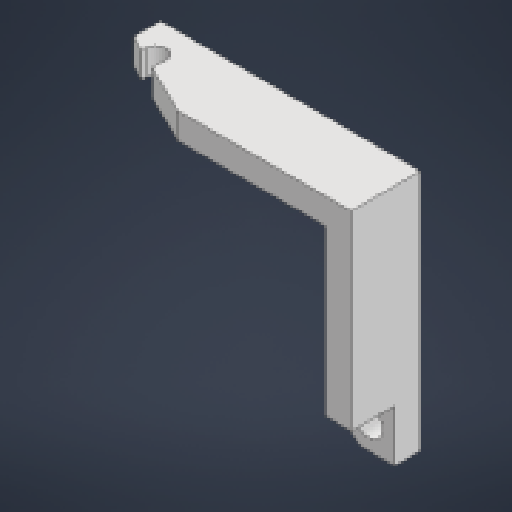
# Autodesk Inventor part: leftfrontwall
Saved by Autodesk Inventor 2026.2 (Build 302298010, 298A)
## iProperties
Created: 2026-09-21
Part Number: leftfrontwall
Material: Generic
Document SubType Name: Modeling
Designer: karol
Density: 1 g/cm^3
Appearance: Default
Author: karol
Autodesk Inventor part; units mm, degrees
ref_plane "YZ Plane" through (0, 0, 0) normal (1, 0, 0) x (0, 1, 0)
ref_plane "XZ Plane" through (0, 0, 0) normal (0, 1, 0) x (-1, 0, 0)
ref_plane "XY Plane" through (0, 0, 0) normal (0, 0, 1) x (1, 0, 0)
sketch "Sketch1" plane through (0, 0, 0) normal (0, 0, 1) x (1, 0, 0)
  line L0 (-58, -60) -> (-60, -60) projected
  line L1 (-60, -60) -> (-60, -39.5) projected
  line L2 (-60, -39.5) -> (-58, -39.5) projected
  line L3 (-58, -39.5) -> (-58, -60) projected
  line L4 (49.6, 30) -> (51.6, 30) projected
  line L5 (51.6, 30) -> (51.6, 9.5) projected
  line L6 (51.6, 9.5) -> (49.6, 9.5) projected
  line L7 (49.6, 9.5) -> (49.6, 30) projected
  line L8 (-58, 39.5) -> (-60, 39.5) projected
  line L9 (-60, 39.5) -> (-60, 60) projected
  line L10 (-60, 60) -> (-58, 60) projected
  line L11 (-58, 60) -> (-58, 39.5) projected
  line L12 (-21.6, -39.5) -> (-19.6, -39.5) projected
  line L13 (-19.6, -39.5) -> (-19.6, -60) projected
  line L14 (-19.6, -60) -> (-21.6, -60) projected
  line L15 (-21.6, -60) -> (-21.6, -39.5) projected
  line L16 (51.6, -30) -> (49.6, -30) projected
  line L17 (49.6, -30) -> (49.6, -9.5) projected
  line L18 (49.6, -9.5) -> (51.6, -9.5) projected
  line L19 (51.6, -9.5) -> (51.6, -30) projected
  line L20 (-21.6, 60) -> (-19.6, 60) projected
  line L21 (-19.6, 60) -> (-19.6, 39.5) projected
  line L22 (-19.6, 39.5) -> (-21.6, 39.5) projected
  line L23 (-21.6, 39.5) -> (-21.6, 60) projected
  line L24 (90, -35) -> (90, 35) projected
  line L25 (90, 35) -> (49.6, 35) projected
  line L26 (49.6, 35) -> (49.6, 60) projected
  line L27 (49.6, 60) -> (90, 60) projected
  line L28 (90, 60) -> (90, 90) projected
  line L29 (90, 90) -> (-19.6, 90) projected
  line L30 (-19.6, 90) -> (-19.6, 65) projected
  line L31 (-19.6, 65) -> (-60, 65) projected
  line L32 (-60, 65) -> (-60, 90) projected
  line L33 (-60, 90) -> (-90, 90) projected
  line L34 (-90, 90) -> (-90, -90) projected
  line L35 (-90, -90) -> (-60, -90) projected
  line L36 (-60, -90) -> (-60, -65) projected
  line L37 (-60, -65) -> (-19.6, -65) projected
  line L38 (-19.6, -65) -> (-19.6, -90) projected
  line L39 (-19.6, -90) -> (90, -90) projected
  line L40 (90, -90) -> (90, -60) projected
  line L41 (90, -60) -> (49.6, -60) projected
  line L42 (49.6, -60) -> (49.6, -35) projected
  line L43 (49.6, -35) -> (90, -35) projected
  line L44 (86, -32) -> (73.8, -32) projected
  line L45 (73.8, -32) -> (73.8, -7.5) projected
  line L46 (73.8, -7.5) -> (86, -7.5) projected
  line L47 (86, -7.5) -> (86, -32) projected
  line L48 (65.8, -32) -> (53.6, -32) projected
  line L49 (53.6, -32) -> (53.6, -7.5) projected
  line L50 (53.6, -7.5) -> (65.8, -7.5) projected
  line L51 (65.8, -7.5) -> (65.8, -32) projected
  line L52 (86, -86) -> (70.6, -86) projected
  line L53 (70.6, -86) -> (70.6, -69.8) projected
  line L54 (70.6, -69.8) -> (86, -69.8) projected
  line L55 (86, -69.8) -> (86, -86) projected
  line L56 (86, 86) -> (86, 69.8) projected
  line L57 (86, 69.8) -> (70.6, 69.8) projected
  line L58 (70.6, 69.8) -> (70.6, 86) projected
  line L59 (70.6, 86) -> (86, 86) projected
  line L60 (73.8, 32) -> (86, 32) projected
  line L61 (86, 32) -> (86, 7.5) projected
  line L62 (86, 7.5) -> (73.8, 7.5) projected
  line L63 (73.8, 7.5) -> (73.8, 32) projected
  line L64 (65.8, 32) -> (65.8, 7.5) projected
  line L65 (65.8, 7.5) -> (53.6, 7.5) projected
  line L66 (53.6, 7.5) -> (53.6, 32) projected
  line L67 (53.6, 32) -> (65.8, 32) projected
  line L68 (-69.6, -87) -> (-85, -87) projected
  line L69 (-85, -87) -> (-85, -70.8) projected
  line L70 (-85, -70.8) -> (-69.6, -70.8) projected
  line L71 (-69.6, -70.8) -> (-69.6, -87) projected
  line L72 (-56, -62) -> (-56, -37.5) projected
  line L73 (-56, -37.5) -> (-43.8, -37.5) projected
  line L74 (-43.8, -37.5) -> (-43.8, -62) projected
  line L75 (-43.8, -62) -> (-56, -62) projected
  line L76 (-56, 62) -> (-43.8, 62) projected
  line L77 (-43.8, 62) -> (-43.8, 37.5) projected
  line L78 (-43.8, 37.5) -> (-56, 37.5) projected
  line L79 (-56, 37.5) -> (-56, 62) projected
  line L80 (-23.6, 62) -> (-23.6, 37.5) projected
  line L81 (-23.6, 37.5) -> (-35.8, 37.5) projected
  line L82 (-35.8, 37.5) -> (-35.8, 62) projected
  line L83 (-35.8, 62) -> (-23.6, 62) projected
  line L84 (-23.6, -62) -> (-35.8, -62) projected
  line L85 (-35.8, -62) -> (-35.8, -37.5) projected
  line L86 (-35.8, -37.5) -> (-23.6, -37.5) projected
  line L87 (-23.6, -37.5) -> (-23.6, -62) projected
  line L88 (-85, 87) -> (-69.6, 87) projected
  line L89 (-69.6, 87) -> (-69.6, 70.8) projected
  line L90 (-69.6, 70.8) -> (-85, 70.8) projected
  line L91 (-85, 70.8) -> (-85, 87) projected
  line L92 (-90, 90) -> (-60, 90)
  line L93 (-60, 90) -> (-60, 87)
  line L94 (-60, 87) -> (-90, 87)
  line L95 (-90, 87) -> (-90, 90)
  line L96 (-90, 90) -> (-60, 90)
  line L97 (-60, 90) -> (-60, 87)
  line L98 (-60, 87) -> (-90, 87)
  line L99 (-90, 87) -> (-90, 90)
  line L100 (-19.6, 65) -> (-60, 65) projected
  line L101 (-60, 65) -> (-60, 68) projected
  line L102 (-60, 68) -> (-63, 68) projected
  line L103 (-63, 62) -> (-16.6, 62) projected
  line L104 (-19.6, 68) -> (-19.6, 65) projected
  line L105 (-60, 87) -> (-63, 87)
  line L106 (-63, 87) -> (-63, 68)
  line L107 (-63, 68) -> (-60, 68)
  line L108 (-60, 68) -> (-60, 87)
  circle A0 centre (-63, -65) radius 1.5 projected
  circle A1 centre (-16.6, -87) radius 1.5 projected
  circle A2 centre (49.6, -87) radius 1.5 projected
  circle A3 centre (46.6, -60) radius 1.5 projected
  circle A4 centre (87, -63) radius 1.5 projected
  circle A5 centre (46.6, -32) radius 1.5 projected
  circle A6 centre (46.6, 32) radius 1.5 projected
  circle A7 centre (87, 63) radius 1.5 projected
  circle A8 centre (46.6, 60) radius 1.5 projected
  circle A9 centre (49.6, 87) radius 1.5 projected
  circle A10 centre (-16.6, 87) radius 1.5 projected
  circle A11 centre (-16.6, 65) radius 1.5 projected
  circle A12 centre (-63, 65) radius 1.5 projected
  arc A13 (-63, 68) -> (-63, 62) centre (-63, 65) ccw projected
  arc A14 (-16.6, 62) -> (-16.6, 68) centre (-16.6, 65) ccw projected
  line L109 (-16.6, 68) -> (-19.6, 68) projected
  line L110 (-76, -39.25) -> (-82, -39.25) projected
  line L111 (-82, -39.25) -> (-82, -20.75) projected
  line L112 (-82, -20.75) -> (-76, -20.75) projected
  line L113 (-76, -20.75) -> (-76, -39.25) projected
  line L114 (-76, 20.75) -> (-82, 20.75) projected
  line L115 (-82, 20.75) -> (-82, 39.25) projected
  line L116 (-82, 39.25) -> (-76, 39.25) projected
  line L117 (-76, 39.25) -> (-76, 20.75) projected
  circle A15 centre (-86.5, -55.7158) radius 1.25 projected
  circle A16 centre (-86.5, 55.8) radius 1.25 projected
  circle A17 centre (-79.5, -5.4579) radius 1.25 projected
  circle A18 centre (-79.5, 5.5421) radius 1.25 projected
  point P0 (0, 0)
  constraints: 24 end point, 6 parallel, 3 horizontal, 3 perpendicular, 2 point on line
extrude "Extrusion1" add sketch "Sketch1" along normal blind 8 contours L102 L106 L94 L32 | L34 L33 L32 L94 L88
sketch "Sketch2" plane through (-63, 68, 0) normal (-1, 0, 0) x (0, 0, 1)
  line L0 (0, 0) -> (3, 0)
  line L1 (3, 0) -> (3, -6)
  line L2 (3, -6) -> (0, -6)
  line L3 (0, -6) -> (0, 0)
  point P0 (0, -68)
  dimension "d2" = 3
  dimension "d3" = 6
  constraints: 8 end point, 2 parallel, 1 horizontal, 1 perpendicular
  measures "d2" distance of L1.end L2.end
  measures "d3" distance of L0.end L1.end
extrude "Extrusion2" add sketch "Sketch2" along normal mid plane 6
sketch "Sketch3" plane through (-66, 62, 3) normal (0, 0, 1) x (1, 0, 0)
  circle A0 centre (3, 3) radius 2 projected
  circle A1 centre (3, 3) radius 1.65
  point P0 (66, -62)
  dimension "d6" = 3.3
  constraints: 1 centre point, 1 coincident
  measures "d6" diameter of A1
extrude "Extrusion3" cut sketch "Sketch3" against normal blind 3 contours A1
sketch "Sketch4" plane through (-90, 90, 0) normal (0, 1, 0) x (1, 0, 0)
  line L0 (0, 0) -> (27, 0) projected
  line L1 (0, 0) -> (0, -3.137)
  line L2 (0, 0) -> (0, -8) projected
  line L3 (0, -3.137) -> (9.9706, -8)
  line L4 (0, -3.137) -> (11.0933, -3.137) construction
  line L5 (30, -8) -> (0, -8) projected
  point P0 (90, 0)
  dimension "d9" = 3.137
  dimension "d10" = 26
  constraints: 6 end point, 2 point on line, 1 equal length, 1 horizontal
  measures "d9" distance of L0.start L1.end
  measures "d10" angle of L3 L4
extrude "Extrusion4" cut sketch "Sketch4" against normal blind 3
fillet "Fillet1" radius 3 2 edges at (-66, 62, 1.5) (-66, 68, 1.5)
sketch "Sketch5" plane through (-90, 90, 0) normal (0, 1, 0) x (1, 0, 0)
  circle A0 centre (3, -3.6) radius 1.2 projected
  line L0 (4.2, -4.8) -> (1.8, -4.8)
  line L1 (1.8, -4.8) -> (1.8, -2.4)
  line L2 (1.8, -2.4) -> (4.2, -2.4)
  line L3 (4.2, -2.4) -> (4.2, -4.8)
  line L4 (4.2, -4.8) -> (1.8, -2.4) construction
  line L5 (1.8, -4.8) -> (4.2, -2.4) construction
  line L6 (4.2, -4.8) -> (4.2, -5.1855)
  line L7 (9.9706, -8) -> (0, -3.137) projected
  line L8 (4.2, -5.1855) -> (3.3204, -4.7564)
  point P0 (90, 0)
  point P1 (4.2, -3.6)
  point P2 (3, -2.4)
  point P3 (3, -4.8)
  point P4 (1.8, -3.6)
  point P5 (3.4097, -4.8)
  point P6 (1.8, -4.0149)
  constraints: 16 end point, 2 midpoint, 2 parallel, 2 point on line, 1 horizontal, 1 perpendicular, 1 vertical, 2 other
extrude "Extrusion5" cut sketch "Sketch5" against normal blind 3 contours L7 A0 | A0 L3 L0 L7 | L0 L6 L7 | L7 L1 A0 picked at (3.1852, -3.7592)
body "Solid1"
